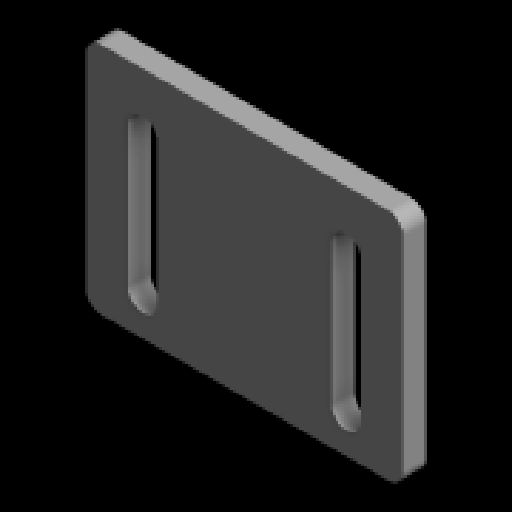
# Autodesk Inventor part: CameraMount
Saved by Autodesk Inventor 2025.2 (Build 292293000, 293)
## iProperties
Created: 2024-12-21
Part Number: CameraMount
Material: Generic
Document SubType Name: Sheet Metal
Designer: valer
Density: 1 g/cm^3
Sheet Metal Rule: Default
Appearance: Default
Author: valer
Autodesk Inventor part; units mm, degrees
ref_plane "YZ Plane" through (0, 0, 0) normal (1, 0, 0) x (0, 1, 0)
ref_plane "XZ Plane" through (0, 0, 0) normal (0, 1, 0) x (-1, 0, 0)
ref_plane "XY Plane" through (0, 0, 0) normal (0, 0, 1) x (1, 0, 0)
sketch "Sketch1" plane through (0, 0, 0) normal (0, 0, 1) x (1, 0, 0)
  line L0 (-29.415, -3) -> (12.585, -3)
  line L1 (12.585, -3) -> (12.585, -34)
  line L2 (12.585, -34) -> (-29.415, -34)
  line L3 (-29.415, -34) -> (-29.415, -3)
  line L4 (-29.6345, -34) -> (12.8045, -34)
  line L5 (-29.415, -3) -> (-15.931, -3)
  line L6 (-8.415, -407.2393) -> (-8.415, 249.8336) construction
  line L7 (-29.415, -18) -> (-29.415, -3) construction
  circle A0 centre (-21.915, -10.5) radius 2 construction
  circle A1 centre (5.085, -10.5) radius 2 construction
  circle A2 centre (-21.915, -29) radius 2.33 construction
  circle A3 centre (5.085, -29) radius 2.33 construction
  line L8 (-21.915, -10.5) -> (5.085, -10.5) construction
  line L9 (-21.915, -29) -> (5.085, -29) construction
  circle A4 centre (-21.915, -10.5) radius 2 construction
  circle A5 centre (5.085, -10.5) radius 2 construction
  circle A6 centre (5.085, -29) radius 2
  circle A7 centre (-21.915, -29) radius 2
  line L10 (-21.915, -10.5) -> (-21.915, -29) construction
  line L11 (-23.915, -10.5) -> (-23.915, -29)
  line L12 (-19.915, -29) -> (-19.915, -10.5)
  arc A8 (-19.915, -10.5) -> (-23.915, -10.5) centre (-21.915, -10.5) ccw
  arc A9 (-23.915, -29) -> (-19.915, -29) centre (-21.915, -29) ccw
  circle A10 centre (-21.915, -10.5) radius 2 construction
  line L13 (7.085, -10.5) -> (7.085, -29)
  line L14 (3.085, -29) -> (3.085, -10.5)
  arc A11 (7.085, -10.5) -> (3.085, -10.5) centre (5.085, -10.5) ccw
  arc A12 (3.085, -29) -> (7.085, -29) centre (5.085, -29) ccw
  point P0 (0, 0)
  point P1 (-8.415, -34)
  point P2 (-21.915, -19.75)
  point P3 (7.085, -29)
extrude "Plate1" add sketch "Sketch1" along normal blind 3
fillet "Fillet1" radius 2 4 edges at (-29.415, -34, 1.5) (12.585, -34, 1.5) (-29.415, -3, 1.5) (12.585, -3, 1.5)
equation "\"d7\" = Thickness"
equation "\"BendRadius\" = Thickness"
equation "\"BendReliefWidth\" = Thickness"
equation "\"BendReliefDepth\" = 0.5 * Thickness"
equation "\"CornerReliefSize\" = 4 * Thickness"
equation "\"MinimumRemnant\" = 2 * Thickness"
equation "\"TransitionRadius\" = BendRadius"
equation "\"JacobiRadiusSize\" = BendRadius"
equation "\"GapSize\" = Thickness"
equation "\"Thickness\" = 3"
body "Solid1"
